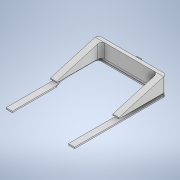
# Autodesk Inventor part: Khay gạt cốc
Saved by Autodesk Inventor 2020 (Build 240168000, 168)
## iProperties
Created: 2022-04-01
Part Number: Khay gạt cốc
Material: Generic
Document SubType Name: Modeling
Designer: PC
Density: 1 g/cm^3
Appearance: Default
Author: PC
Autodesk Inventor part; units mm, degrees
ref_plane "YZ Plane" through (0, 0, 0) normal (1, 0, 0) x (0, 1, 0)
ref_plane "XZ Plane" through (0, 0, 0) normal (0, 1, 0) x (-1, 0, 0)
ref_plane "XY Plane" through (0, 0, 0) normal (0, 0, 1) x (1, 0, 0)
sketch "Sketch1" plane through (0, 0, 0) normal (0, 1, 0) x (-1, 0, 0)
  line L0 (50, -60) -> (-50, -60)
  line L1 (-50, -60) -> (-50, 60)
  line L2 (-50, 60) -> (50, 60)
  line L3 (50, 60) -> (50, -60)
  line L4 (50, -60) -> (-50, 60) construction
  line L5 (-50, -60) -> (50, 60) construction
  point P0 (0, 0)
  dimension "d0" = 100
  dimension "d1" = 120
  constraints: 12 end point, 2 midpoint, 2 parallel, 1 horizontal, 1 perpendicular
  measures "d0" distance of L1.end L2.end
  measures "d1" distance of L0.end L1.end
extrude "Extrusion1" add sketch "Sketch1" along normal blind 26
sketch "Sketch2" plane through (0, 26, 0) normal (0, 1, 0) x (1, 0, 0)
  line L0 (-41, -60) -> (41, -60)
  line L1 (-50, -60) -> (50, -60) projected
  line L2 (41, -60) -> (41, -4.7988)
  line L3 (50, 60) -> (-50, 60) projected
  line L4 (-41, -60) -> (-41, 55)
  line L5 (-41, 55) -> (41, 55)
  line L6 (41, 55) -> (41, -4.7988)
  point P0 (0, 0)
  dimension "d23" = 115
  constraints: 10 end point, 4 perpendicular, 1 point on line
  measures "d23" distance of L0.start L4.end
extrude "Extrusion2" cut sketch "Sketch2" against normal through all
sketch "Sketch11" plane through (0, 0, 0) normal (0, -1, 0) x (1, 0, 0)
  arc A0 (46, -10.5) -> (-46, -10.5) centre (0, -10.5) ccw
  line L0 (41, -55) -> (-41, -55) projected
  line L1 (-46, -10.5) -> (46, -10.5)
  line L2 (46, -10.5) -> (46, -55)
  line L3 (46, -55) -> (-46, -55)
  line L4 (-46, -55) -> (-46, -10.5)
  point P0 (0, 0)
  dimension "d24" = 92
  dimension "d25" = 44.5
  constraints: 8 end point, 2 parallel, 2 point on circle, 1 centre point, 1 horizontal, 1 perpendicular
  measures "d24" diameter of A0
  measures "d25" distance from line of A0.centre L0
extrude "Extrusion7" cut sketch "Sketch11" against normal blind 5.4
sketch "Sketch13" plane through (-41, 26, 60) normal (1, 0, 0) x (0, 0, -1)
  line L0 (0, -26) -> (0, 0) projected
  line L1 (0, -24) -> (115.5309, -24)
  line L2 (115.5309, -24) -> (115.5309, -20.6)
  line L3 (115.5309, -20.6) -> (0, -20.6)
  line L4 (0, -20.6) -> (0, -24)
  line L5 (49.6433, -26) -> (0, -26) projected
  point P0 (60, -26)
  point P1 (0, -20.6)
  dimension "d48" = 115.5309
  dimension "d49" = 3.4
  dimension "d50" = 2
  constraints: 8 end point, 2 parallel, 1 horizontal, 1 perpendicular, 1 point on line
  measures "d48" distance of L2.end L3.end
  measures "d49" distance of L1.end L2.end
  measures "d50" distance between parallel lines of L5 L1
extrude "Extrusion8" cut sketch "Sketch13" against normal through all both and the other way through all
sketch "Sketch14" plane through (-41, 26, 60) normal (1, 0, 0) x (0, 0, -1)
  line L0 (0, -20.6) -> (0, 0) projected
  line L1 (0, 0) -> (49.643, 0)
  line L2 (49.643, 0) -> (49.643, -20.6)
  line L3 (49.643, -20.6) -> (0, -20.6)
  line L4 (0, -20.6) -> (0, 0)
  point P0 (60, -26)
  dimension "d51" = 20.6
  dimension "d52" = 49.643
  constraints: 8 end point, 2 parallel, 1 horizontal, 1 perpendicular
  measures "d51" distance of L1.end L2.end
  measures "d52" distance of L2.end L3.end
extrude "Extrusion9" cut sketch "Sketch14" along normal through all both and the other way through all
sketch "Sketch15" plane through (0, 0, 0) normal (1, 0, 0) x (0, 1, 0)
  line L0 (26, -55) -> (5.4, -55) projected
  line L1 (7, 10.357) -> (26, -55)
  line L2 (26, -55) -> (26, 10.357)
  line L3 (26, 10.357) -> (7, 10.357)
  point P0 (0, 0)
  dimension "d53" = 65.357
  dimension "d54" = 19
  constraints: 6 end point, 2 perpendicular
  measures "d53" distance of L0.start L2.end
  measures "d54" distance of L2.end L1.start
extrude "Extrusion10" cut sketch "Sketch15" against normal through all both and the other way through all
fillet "Fillet1" radius 5 4 edges at (-41, 15.7, -55) (50, 13, -60) (-50, 13, -60) (41, 15.7, -55)
fillet "Fillet2" radius 5 2 edges at (-46, 1, -55) (46, 1, -55)
sketch "Sketch16" plane through (45, 0, -60) normal (0, 0, -1) x (-1, 0, 0)
  line L0 (45, 0) -> (45, 26)
  line L1 (81, 26) -> (9, 26) projected
  line L2 (40.8, 17.5345) -> (49.2, 17.5345)
  line L3 (49.2, 17.5345) -> (49.2, 14.5345)
  line L4 (49.2, 14.5345) -> (40.8, 14.5345)
  line L5 (40.8, 14.5345) -> (40.8, 17.5345)
  line L6 (40.8, 17.5345) -> (49.2, 14.5345) construction
  line L7 (49.2, 17.5345) -> (40.8, 14.5345) construction
  point P0 (45, 16.0345)
  dimension "d38" = 8.4
  dimension "d39" = 3
  constraints: 14 end point, 3 midpoint, 2 parallel, 1 horizontal, 1 perpendicular, 1 point on line
  measures "d38" distance of L3.end L4.end
  measures "d39" distance of L2.end L3.end
extrude "Extrusion11" add sketch "Sketch16" along normal blind 10
sketch "Sketch17" plane through (-4.2, 17.5345, -60) normal (0, 1, 0) x (1, 0, 0)
  circle A0 centre (4.2, 5.8) radius 2.7
  line L0 (0, 0) -> (0, 10) projected
  line L1 (0, 10) -> (8.4, 10) projected
  point P0 (4.2, -60)
  dimension "d42" = 5.4
  dimension "d43" = 4.2
  dimension "d44" = 4.2
  constraints: 1 centre point
  measures "d42" diameter of A0
  measures "d43" distance from line of L0 A0.centre
  measures "d44" distance from line of L1 A0.centre
extrude "Extrusion12" cut sketch "Sketch17" against normal through all
fillet "Fillet5" radius 2 2 edges at (-4.2, 16.0345, -70) (4.2, 16.0345, -70)
sketch "Sketch18" plane through (45, 0, -60) normal (0, 0, -1) x (-1, 0, 0)
  point P0 (45, 0)
sketch "Sketch19" plane through (-50, 5.4, -55) normal (-1, 0, 0) x (0, 0, 1)
  point P0 (55, -5.4)
sketch "Sketch20" plane through (-50, 0, 60) normal (0, 0, 1) x (1, 0, 0)
  line L0 (9, 2) -> (0, 2) projected
  line L1 (0, 0) -> (9, 0) projected
  line L2 (0, 2) -> (9, 2)
  line L3 (9, 2) -> (9, 0)
  line L4 (9, 0) -> (0, 0)
  line L5 (0, 0) -> (0, 2)
  line L6 (100, 0) -> (95, 0) projected
  line L7 (100, 2) -> (91, 2) projected
  line L8 (100, 0) -> (91, 0)
  line L9 (91, 0) -> (91, 2)
  line L10 (91, 2) -> (100, 2)
  line L11 (100, 2) -> (100, 0)
  point P0 (50, 0)
  constraints: 16 end point, 4 parallel, 2 horizontal, 2 perpendicular
extrude "Extrusion13" add sketch "Sketch20" along normal blind 15
body "Solid1"
